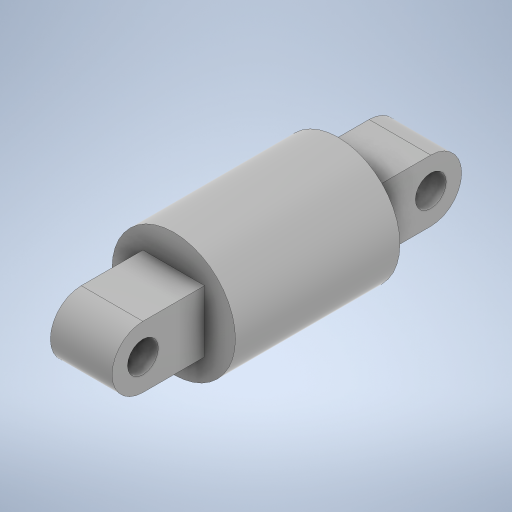
# Autodesk Inventor part: Neck
Saved by Autodesk Inventor 2024 (Build 280153000, 153)
## iProperties
Created: 2023-06-07
Part Number: Neck
Material: Generic
Document SubType Name: Modeling
Designer: Samyak Gosalia
Density: 1 g/cm^3
Appearance: Default
Author: Samyak Gosalia
Autodesk Inventor part; units mm, degrees
ref_plane "YZ Plane" through (0, 0, 0) normal (1, 0, 0) x (0, 1, 0)
ref_plane "XZ Plane" through (0, 0, 0) normal (0, 1, 0) x (-1, 0, 0)
ref_plane "XY Plane" through (0, 0, 0) normal (0, 0, 1) x (1, 0, 0)
sketch "Sketch1" plane through (0, 0, 0) normal (0, 0, 1) x (1, 0, 0)
  circle A0 centre (0, 0) radius 15
  dimension "d0" = 30
  constraints: 1 centre point, 1 coincident
  measures "d0" diameter of A0
extrude "Extrusion1" add sketch "Sketch1" along normal blind 40
sketch "Sketch2" plane through (0, 0, 40) normal (0, 0, 1) x (1, 0, 0)
  line L0 (7.5, 7.5) -> (7.5, -7.5)
  line L1 (-7.5, 7.5) -> (-7.5, -7.5)
  line L2 (-7.5, 7.5) -> (7.5, 7.5)
  line L3 (-7.5, -7.5) -> (7.5, -7.5)
  point P0 (0, 0)
  dimension "d3" = 7.5
  dimension "d4" = 7.5
  dimension "d5" = 7.5
  dimension "d6" = 7.5
  constraints: 8 end point, 2 vertical, 1 horizontal, 1 perpendicular
  measures "d3" distance from line of L1 point (0, 0)
  measures "d4" distance from line of L0 point (0, 0)
  measures "d5" distance from line of point (0, 0) L2
  measures "d6" distance from line of L3 point (0, 0)
extrude "Extrusion2" add sketch "Sketch2" along normal blind 22.5
fillet "Fillet1" radius 7.5 2 edges at (0, 7.5, 62.5) (0, -7.5, 62.5)
sketch "Sketch3" plane through (0, 0, 0) normal (1, 0, 0) x (0, 1, 0)
  line L0 (7.5, 40) -> (7.5, 55) projected
  line L1 (-7.5, 40) -> (-7.5, 55) projected
  line L2 (7.5, 55) -> (-7.5, 55) construction
  circle A0 centre (0, 55) radius 3.75
  point P0 (0, 0)
  dimension "d10" = 7.5
  constraints: 2 end point, 1 centre point, 1 horizontal, 1 midpoint
  measures "d10" diameter of A0
extrude "Extrusion3" cut sketch "Sketch3" along normal through all both and the other way through all
sketch "Sketch4" plane through (0, 0, 0) normal (0, 0, -1) x (-1, 0, 0)
  line L0 (-7.5, 7.5) -> (7.5, 7.5)
  line L1 (7.5, 7.5) -> (7.5, -7.5)
  line L2 (7.5, -7.5) -> (-7.5, -7.5)
  line L3 (-7.5, -7.5) -> (-7.5, 7.5)
  line L4 (-7.5, 7.5) -> (7.5, -7.5) construction
  line L5 (7.5, 7.5) -> (-7.5, -7.5) construction
  point P0 (0, 0)
  dimension "d13" = 15
  dimension "d14" = 15
  constraints: 12 end point, 2 midpoint, 2 parallel, 1 horizontal, 1 perpendicular
  measures "d13" distance of L1.end L2.end
  measures "d14" distance of L0.end L1.end
extrude "Extrusion4" add sketch "Sketch4" along normal blind 22.5
fillet "Fillet2" radius 7.5 2 edges at (0, 7.5, -22.5) (0, -7.5, -22.5)
sketch "Sketch5" plane through (7.5, -7.5, 0) normal (1, 0, 0) x (0, 0, -1)
  line L0 (0, 15) -> (15, 15) projected
  line L1 (0, 0) -> (15, 0) projected
  line L2 (15, 15) -> (15, 0) construction
  circle A0 centre (15, 7.5) radius 3.75
  point P0 (0, 7.5)
  dimension "d18" = 7.5
  constraints: 2 end point, 1 centre point, 1 midpoint, 1 vertical
  measures "d18" diameter of A0
extrude "Extrusion5" cut sketch "Sketch5" against normal through all
body "Solid1"
